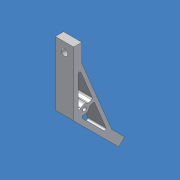
# Autodesk Inventor part: HBL135TS6hbl45ts6
Saved by Autodesk Inventor 2014 SP1 (Build 180222100, 222)
## iProperties
Category: PARTsolutions
Created: 2015-02-11
Part Number: HBL135TS6hbl45ts6
Catalog Web Link: www.cadenas.de
Description: HBL45TS6, HBL45TD6, HBL135TS6, HBL135TD6 - Brackets with Angle 45/135 Deg.
Document SubType Name: Modeling
Designer: PARTsolutions
Material: Generic
Density: 1 g/cm^3
Appearance: RGB(192,192,192)
NB: HBL135TS6hbl45ts6
NN: HBL45TS6, HBL45TD6, HBL135TS6, HBL135TD6
NT: Brackets with Angle 45/135 Deg.
NBSYN: $PN.hbl45ts6
LINA: HBL135TS6hbl45ts6
PN: HBL135TS6
TP: HBL135TS6
MAT: JIS-A6N01SS-T5
ST: Anodizing
TYPE: HBL135TS6
FEAT: Brackets with Angle 135 Deg.
SLOT: Slot Width 8 Frame
MASS: 68
AB: CBM6-15
NOB: 2
AN: HNTT6-6
NON: 2
AL: 1176
W: 20
DIA: 7.0
ALT1OPT: '','w/o C (Mounting Holes for Cover)','-C','with C (Mounting Holes for Cover)'
VER: 6
DIS: 0.000
VERS: 7.000
KT: 7
SUPPLIER: Misumi
ARTICLENO: HBL135TS6hbl45ts6
BOMINFO: HBL135TS6hbl45ts6
CREATOR: CADENAS GmbH
PSOL_IDENT_0: {\\10.0.0.236\data_v8\23d-libs\misumi\metric\38_al_extrusions_blackets\6\hbl45ts6.prj},220 {VTYP=3D}
PSOL_IDENT_1: ,{NB=HBL135TS6hbl45ts6},{LINA=HBL135TS6hbl45ts6},{NN=HBL45TS6, HBL45TD6, HBL135TS6, HBL135TD6},{DATE
PSOL_IDENT_2: =19.11.2014 02:28:17},{GEOMDATE=12.03.2009 12:55:00},{VERSION=},{LINEID=240},{LINESUBID=-1},{WBVAR=A
PSOL_IDENT_3: LT1,ALT3}  {NB=HBL135TS6hbl45ts6},{LINA=HBL135TS6hbl45ts6},{KT=7},{PN=HBL135TS6},{TP=HBL135TS6},{MAT
PSOL_IDENT_4: =JIS-A6N01SS-T5},{ST=Anodizing},{TYPE=HBL135TS6},{FEAT=Brackets with Angle 135 Deg.},{SLOT=Slot Widt
PSOL_IDENT_5: h 8 Frame},{ALT1=},{ALT3=},{MASS=68},{AB=CBM6-15},{NOB=2},{AN=HNTT6-6},{NON=2},{AL=1176},{W=20},{DIA
PSOL_IDENT_6: =7.0},{ALT1OPT='','w/o C (Mounting Holes for Cover)','-C','with C (Mounting Holes for Cover)'},{VER=
PSOL_IDENT_7: 6},{DIS=0.000},{VERS=7.000}
Title: HBL135TS6hbl45ts6
Author: Cadenas PARTsolutions
Comments: Brackets with Angle 45/135 Deg.
Autodesk Inventor part; units mm, degrees
sketch "Sketch_8" plane through (0, 0, 0) normal (1, 0, 0) x (0, 1, 0)
  line L0 (0, 70) -> (0, 0)
  line L1 (0, 0) -> (49.4975, -49.4975)
  line L2 (49.4975, -49.4975) -> (55.8614, -43.1335)
  line L3 (55.8614, -43.1335) -> (41.7193, -28.9914)
  line L4 (41.7193, -28.9914) -> (9, 49.9914)
  line L5 (9, 49.9914) -> (9, 70)
  line L6 (9, 70) -> (0, 70)
  arc A0 (23.0035, 5.74) -> (21.0437, 6.5518) centre (21.6177, 5.166) ccw
  line L7 (21.0437, 6.5518) -> (17.935, 5.2641)
  arc A1 (17.935, 5.2641) -> (17.0297, 4.1265) centre (18.509, 3.8783) ccw
  arc A2 (10.9882, -0.0281) -> (17.0297, 4.1265) centre (12, 4.9706) ccw
  arc A3 (10.9882, -0.0281) -> (9.63, -2.5589) centre (10.6906, -1.4983) ccw
  line L8 (9.63, -2.5589) -> (32.996, -25.9249)
  arc A4 (32.996, -25.9249) -> (35.4424, -24.2902) centre (34.0566, -24.8642) ccw
  line L9 (35.4424, -24.2902) -> (23.0035, 5.74)
  circle A5 centre (12, 4.9706) radius 2.1
  arc A6 (7.8859, 42.2372) -> (5.0029, 41.7559) centre (6.5, 41.6633) ccw
  line L10 (5.0029, 41.7559) -> (5, 8.619)
  arc A7 (5, 8.619) -> (7.7564, 7.7993) centre (6.5, 8.6189) ccw
  arc A8 (14.9597, 9.1239) -> (7.7564, 7.7993) centre (12, 4.9705) ccw
  arc A9 (14.9597, 9.1239) -> (16.4042, 8.9596) centre (15.8302, 10.3455) ccw
  line L11 (16.4042, 8.9596) -> (19.5129, 10.2473)
  arc A10 (19.5129, 10.2473) -> (20.3596, 12.1145) centre (18.9389, 11.6331) ccw
  line L12 (20.3596, 12.1145) -> (7.8859, 42.2372)
  constraints: 26 end point, 20 point on circle, 11 centre point
extrude "Extrusion1" add sketch "Sketch_8" along normal mid plane 20
sketch "Sketch_3" plane through (0, 0, 0) normal (0, 1, 0) x (-1, 0, 0)
  circle A0 centre (0, 60) radius 3.5
  constraints: 1 centre point
extrude "Extrusion2" cut sketch "Sketch_3" along normal blind 9
sketch "Sketch_9" plane through (0, 0, 0) normal (1, 0, 0) x (0, 1, 0)
  line L0 (42.4264, -42.4264) -> (48.7904, -36.0624)
  line L1 (48.7904, -36.0624) -> (51.2652, -38.5373)
  line L2 (51.2652, -38.5373) -> (44.9013, -44.9013)
  line L3 (44.9013, -44.9013) -> (42.4264, -42.4264)
  line L4 (42.4264, -42.4264) -> (48.7904, -36.0624)
  constraints: 10 end point
revolve "Revolution1" cut sketch "Sketch_9" angle 360 about axis through (0, 42.4264, -42.4264) along (0, -0.7071, -0.7071)
ref_plane "bracket_to_dummy_XY" through (0, 0, 0) normal (0, 1, 0) x (1, 0, 0)
ref_plane "bracket_to_dummy_YZ" through (0, 0, 0) normal (1, 0, 0) x (0, 0, -1)
ref_plane "bracket_to_dummy_ZX" through (0, 0, 0) normal (0, 0, -1) x (0, 1, 0)
ref_plane "1_to_bolt_XY" through (0, 9, 60) normal (0, 1, 0) x (1, 0, 0)
ref_plane "1_to_bolt_YZ" through (0, 9, 60) normal (1, 0, 0) x (0, 0, -1)
ref_plane "1_to_bolt_ZX" through (0, 9, 60) normal (0, 0, -1) x (0, 1, 0)
ref_plane "6_to_bolt_XY" through (0, 48.7904, -36.0624) normal (0, 0.7071, 0.7071) x (0, 0.7071, -0.7071)
ref_plane "6_to_bolt_YZ" through (0, 48.7904, -36.0624) normal (0, 0.7071, -0.7071) x (-1, 0, 0)
ref_plane "6_to_bolt_ZX" through (0, 48.7904, -36.0624) normal (-1, 0, 0) x (0, 0.7071, 0.7071)
ref_plane "7_to_bolt_XY" through (30, 48.7904, -36.0624) normal (0, 0.7071, 0.7071) x (0, 0.7071, -0.7071)
ref_plane "7_to_bolt_YZ" through (30, 48.7904, -36.0624) normal (0, 0.7071, -0.7071) x (-1, 0, 0)
ref_plane "7_to_bolt_ZX" through (30, 48.7904, -36.0624) normal (-1, 0, 0) x (0, 0.7071, 0.7071)
ref_plane "8_to_bolt_XY" through (0, 9, 60) normal (0, 1, 0) x (0, 0, -1)
ref_plane "8_to_bolt_YZ" through (0, 9, 60) normal (0, 0, -1) x (-1, 0, 0)
ref_plane "8_to_bolt_ZX" through (0, 9, 60) normal (-1, 0, 0) x (0, 1, 0)
ref_plane "9_to_bolt_XY" through (30, 9, 60) normal (0, 1, 0) x (0, 0, -1)
ref_plane "9_to_bolt_YZ" through (30, 9, 60) normal (0, 0, -1) x (-1, 0, 0)
ref_plane "9_to_bolt_ZX" through (30, 9, 60) normal (-1, 0, 0) x (0, 1, 0)
body "Solid1"
